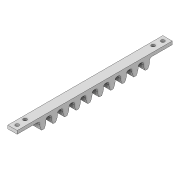
# Autodesk Inventor part: rack6mm-v2-bottom
Saved by Autodesk Inventor 2020 (Build 240168000, 168)
## iProperties
Created: 2021-06-14
Part Number: rack6mm-v2-bottom
Material: Generic
Document SubType Name: Modeling
Designer: Aidan Lee
Density: 1 g/cm^3
Appearance: Default
Author: Aidan Lee
Autodesk Inventor part; units mm, degrees
ref_plane "YZ Plane" through (0, 0, 0) normal (1, 0, 0) x (0, 1, 0)
sketch "Sketch2" plane through (0, 0, 0) normal (0, 0, 1) x (1, 0, 0)
  line L0 (-32.0857, 0) -> (0, 0)
  line L1 (0, 0) -> (0, 19.635)
  line L2 (0, 19.635) -> (-32.0857, 19.635)
  spline S0 degree 3 poles (-32.0857, 19.635) (-32.0786, 19.6019) (-32.0585, 19.4984) (-32.0378, 19.3226) (-32.0222, 19.1083) (-32.0293, 18.8935) (-32.0484, 18.6795) (-32.102, 18.3981) (-32.1765, 18.0482) (-32.2416, 17.6965) (-32.2997, 17.416) (-32.364, 17.211) (-32.4396, 17.0099) (-32.536, 16.8179) (-32.6409, 16.6304) (-32.7641, 16.4543) (-32.8983, 16.2866) (-33.043, 16.1278) (-33.201, 15.9822) (-33.3669, 15.8459) (-33.5414, 15.7205) (-33.7857, 15.5713) (-34.1055, 15.4094) (-34.509, 15.2608) (-34.9249, 15.1525) (-35.3479, 15.078) (-35.7753, 15.0341) (-36.2047, 15.0215) (-36.6341, 15.0313) (-37.0623, 15.0646) (-37.3462, 15.1014) (-37.4881, 15.1198) knots -0.847201 -0.847201 -0.847201 -0.847201 -0.83705 -0.815587 -0.794126 -0.772659 -0.751201 -0.729734 -0.686802 -0.64387 -0.622403 -0.600945 -0.579478 -0.558017 -0.536554 -0.515088 -0.49363 -0.472163 -0.450698 -0.429238 -0.407769 -0.386302 -0.343394 -0.300476 -0.257562 -0.214646 -0.17172 -0.12879 -0.085861 -0.04293 0 0 0 0
  spline S1 degree 3 poles (-37.4881, 15.1198) (-37.594, 15.1249) (-37.8057, 15.1352) (-38.2295, 15.119) (-38.7575, 15.0717) (-39.3865, 14.9771) (-40.0103, 14.8535) (-40.6285, 14.7043) (-41.2408, 14.5326) (-41.847, 14.3405) (-42.4469, 14.1297) (-43.0405, 13.9015) (-43.6276, 13.6572) (-44.2081, 13.3977) (-44.782, 13.1239) (-45.3493, 12.8367) (-45.9097, 12.5363) (-46.4639, 12.2246) (-46.8275, 12.0066) (-47.0092, 11.8976) knots -1.017256 -1.017256 -1.017256 -1.017256 -0.985476 -0.953687 -0.890117 -0.826542 -0.762964 -0.699386 -0.635807 -0.572227 -0.508647 -0.445066 -0.381486 -0.317905 -0.254324 -0.190743 -0.127162 -0.063581 0 0 0 0
  arc A0 (-47.0092, 11.8976) -> (-47.0092, 7.7374) centre (9.2023, 9.8175) ccw
  spline S2 degree 3 poles (-47.0092, 7.7374) (-46.8275, 7.6284) (-46.4639, 7.4104) (-45.9097, 7.0987) (-45.3493, 6.7983) (-44.782, 6.5111) (-44.2081, 6.2373) (-43.6276, 5.9778) (-43.0405, 5.7335) (-42.4469, 5.5053) (-41.847, 5.2945) (-41.2408, 5.1024) (-40.6285, 4.9307) (-40.0103, 4.7815) (-39.3865, 4.6579) (-38.7575, 4.5633) (-38.2295, 4.516) (-37.8057, 4.4998) (-37.594, 4.5101) (-37.4881, 4.5152) knots -1.017256 -1.017256 -1.017256 -1.017256 -0.953675 -0.890094 -0.826513 -0.762932 -0.699351 -0.63577 -0.572189 -0.508609 -0.445029 -0.381449 -0.31787 -0.254291 -0.190714 -0.127139 -0.063568 -0.03178 0 0 0 0
  spline S3 degree 3 poles (-37.4881, 4.5152) (-37.3462, 4.5336) (-37.0623, 4.5704) (-36.6341, 4.6037) (-36.2047, 4.6135) (-35.7753, 4.6009) (-35.3479, 4.557) (-34.9249, 4.4825) (-34.509, 4.3742) (-34.1055, 4.2256) (-33.7857, 4.0637) (-33.5414, 3.9145) (-33.3669, 3.7891) (-33.201, 3.6528) (-33.043, 3.5072) (-32.8983, 3.3484) (-32.7641, 3.1807) (-32.6409, 3.0046) (-32.536, 2.8171) (-32.4396, 2.6251) (-32.364, 2.424) (-32.2997, 2.219) (-32.2416, 1.9385) (-32.1765, 1.5868) (-32.102, 1.2369) (-32.0484, 0.9555) (-32.0293, 0.7415) (-32.0222, 0.5267) (-32.0378, 0.3124) (-32.0585, 0.1366) (-32.0786, 0.0331) (-32.0857, 0) knots -1.373604 -1.373604 -1.373604 -1.373604 -1.330674 -1.287743 -1.244814 -1.201884 -1.158958 -1.116042 -1.073128 -1.03021 -0.987302 -0.965835 -0.944366 -0.922906 -0.901441 -0.879974 -0.858516 -0.83705 -0.815587 -0.794126 -0.772659 -0.751201 -0.729734 -0.686802 -0.64387 -0.622403 -0.600945 -0.579478 -0.558017 -0.536554 -0.526403 -0.526403 -0.526403 -0.526403
  constraints: 6 end point, 2 centre point, 2 point on circle, 16 other
extrude "Extrusion1" add sketch "Sketch2" along normal blind 16
pattern_linear "Rectangular Pattern1" count 10 spacing 19.635 along (0, 1, 0) of "Extrusion1"
sketch "Sketch5" plane through (-32.0857, 0, 0) normal (0, -1, 0) x (1, 0, 0)
  line L0 (32.0857, 0) -> (32.0857, 16) projected
  line L1 (0, 16) -> (32.0857, 16) projected
  line L2 (0, 0) -> (32.0857, 0) projected
  line L3 (0, 0) -> (0, 16) projected
  line L4 (0, 16) -> (8, 16)
  line L5 (8, 16) -> (8, 0) construction
  line L6 (8, 0) -> (0, 0)
  line L7 (0, 0) -> (0, 16)
  line L8 (8, 16) -> (10.5, 16)
  line L9 (10.5, 16) -> (10.5, 10.5)
  line L10 (10.5, 10.5) -> (8, 10.5)
  line L11 (8, 10.5) -> (8, 16) construction
  line L12 (8, 2.5) -> (10.5, 2.5)
  line L13 (10.5, 2.5) -> (10.5, 0)
  line L14 (10.5, 0) -> (8, 0)
  line L15 (8, 0) -> (8, 2.5) construction
  line L16 (8, 9.5) -> (37, 9.5) construction
  line L17 (37, 9.5) -> (37, 3.5) construction
  line L18 (37, 3.5) -> (8, 3.5) construction
  line L19 (8, 3.5) -> (8, 9.5) construction
  line L20 (8, 10.5) -> (8, 2.5)
  line L21 (34.5, 15.5) -> (10.5, 15.5) construction
  line L22 (10.5, 15.5) -> (10.5, 0.5) construction
  line L23 (10.5, 0.5) -> (34.5, 0.5) construction
  line L24 (34.5, 0.5) -> (34.5, 15.5) construction
  line L25 (41.5759, 16) -> (41.5759, 15.5) construction
  line L26 (41.5759, 0.5) -> (41.5759, 0) construction
  line L27 (25.6, 16.05) -> (19.4, 16.05) construction
  line L28 (19.4, -0.05) -> (25.6, -0.05) construction
  line L29 (25.6, -0.05) -> (25.6, 0.5) construction
  line L30 (25.6, 15.5) -> (25.6, 16.05) construction
  line L31 (19.4, 16.05) -> (19.4, 15.5) construction
  line L32 (19.4, 0.5) -> (19.4, -0.05) construction
  line L33 (25.6, 0.5) -> (25.6, 15.5) construction
  line L34 (19.4, 15.5) -> (19.4, 0.5) construction
  point P0 (9.25, 10.5)
  point P1 (9.25, 2.5)
  point P2 (8, 6.5)
  point P3 (8, 6.5)
  point P4 (22.5, 15.5)
  point P5 (22.5, 9.5)
  point P6 (22.5, -0.05)
  dimension "d15" = 8
  dimension "d16" = 8
  dimension "d18" = 6
  dimension "d19" = 29
  dimension "d20" = 24
  dimension "d21" = 6
  dimension "d22" = 3
  dimension "d23" = 2.5
  dimension "d24" = 2.5
  dimension "d30" = 5.5
  dimension "d31" = 2.5
  dimension "d64" = 6.2
  dimension "d65" = 16.1
  constraints: 62 end point, 16 parallel, 14 point on line, 7 midpoint, 7 perpendicular, 6 horizontal, 5 collinear, 3 vertical, 2 horizontal alignment, 2 vertical alignment, 1 coincident
  measures "d15" distance between parallel lines of L3 L5
  measures "d16" distance between parallel lines of L12 L10
  measures "d18" distance of L16.end L17.end
  measures "d19" distance of L16.start L16.end
  measures "d20" distance of L21.start L21.end
  measures "d21" distance between parallel lines of L16 L21
  measures "d22" distance between parallel lines of L23 L18
  measures "d23" distance between parallel lines of L5 L22
  measures "d24" distance between parallel lines of L11 L9
  measures "d30" distance of L8.end L9.end
  measures "d31" distance of L12.end L13.end
  measures "d64" distance of L27.start L27.end
  measures "d65" distance between parallel lines of L28 L27
extrude "Extrusion3" cut sketch "Sketch5" against normal through all contours L2 L13 L12 L20 L10 L9 L1 L0
sketch "Measurements" plane through (0, 0, 0) normal (0, 0, -1) x (-1, 0, 0)
  line L0 (41.7977, 19.635) -> (70.5831, 19.635) construction
  line L1 (141.7977, 176.7146) -> (141.7977, 118.484) construction
  line L2 (21.5857, 196.35) -> (21.5857, 0) projected
  line L3 (32.0857, 0) -> (21.5857, 0) projected
  circle A0 centre (91.7977, 19.635) radius 50 construction
  line L4 (41.7977, -40.4843) -> (41.7977, 79.7543) construction
  line L5 (41.7977, 19.635) -> (141.7977, 19.635) construction
  line L6 (141.7977, 19.635) -> (141.7977, 176.7146) construction
  arc A1 (41.7977, 19.635) -> (141.7977, 176.7146) centre (-31.5724, 176.7146) ccw construction
  circle A2 centre (91.7977, 176.7146) radius 50 construction
  line L7 (-14.9143, 139.9646) -> (32.0857, 139.9646) construction
  line L8 (32.0857, 139.9646) -> (32.0857, 213.4646) construction
  line L9 (32.0857, 213.4646) -> (-14.9143, 213.4646) construction
  line L10 (-14.9143, 213.4646) -> (-14.9143, 139.9646) construction
  circle A3 centre (91.7977, 176.7146) radius 5 construction
  line L11 (32.0857, 139.9646) -> (96.4406, 164.572) construction
  arc A4 (96.4406, 164.572) -> (96.4406, 188.8572) centre (91.7977, 176.7146) ccw construction
  line L12 (96.4406, 188.8572) -> (32.0857, 213.4646) construction
  line L13 (-14.9143, -17.115) -> (32.0857, -17.115) construction
  line L14 (32.0857, -17.115) -> (32.0857, 56.385) construction
  line L15 (32.0857, 56.385) -> (-14.9143, 56.385) construction
  line L16 (-14.9143, 56.385) -> (-14.9143, -17.115) construction
  circle A5 centre (91.7977, 19.635) radius 5 construction
  line L17 (32.0857, -17.115) -> (96.4406, 7.4924) construction
  arc A6 (96.4406, 7.4924) -> (96.4406, 31.7776) centre (91.7977, 19.635) ccw construction
  line L18 (96.4406, 31.7776) -> (32.0857, 56.385) construction
  line L19 (96.7977, 176.7146) -> (96.7977, 157.197) construction
  line L20 (96.7977, 19.635) -> (96.7977, 0.1424) construction
  circle A7 centre (9.5857, 201.4646) radius 14.5 construction
  line L21 (-14.9143, 176.7146) -> (-21.6792, 176.7146)
  circle A8 centre (9.5857, 151.9646) radius 14.5 construction
  point P0 (0, 0)
  point P1 (32.0857, 176.7146)
  point P2 (104.7977, 176.7146)
  point P3 (104.7977, 19.635)
  point P4 (32.0857, 19.635)
  dimension "d43" = 10
  dimension "d32" = 100
  dimension "d33" = 157.0796
  dimension "d34" = 59.712
  dimension "d36" = 73.5
  dimension "d37" = 47
  dimension "d38" = 73.5
  dimension "d39" = 47
  dimension "d41" = 8
  dimension "d44" = 17.115
  dimension "d66" = 29
  dimension "d67" = 12
  dimension "d68" = 24.5
  constraints: 40 end point, 11 point on circle, 9 vertical alignment, 7 centre point, 7 tangent, 6 parallel, 5 horizontal alignment, 5 midpoint, 5 perpendicular, 4 coincident, 4 vertical, 3 horizontal, 1 point on line, 1 symmetric about line, 5 other
  measures "d32" diameter of A0
  measures "d33" distance of L5.end L1.start
  measures "d34" horizontal distance of L3.start A0.centre
  measures "d36" distance of L9.end L7.start
  measures "d37" distance of L7.start L7.end
  measures "d38" distance of L16.start L13.start
  measures "d39" distance of L13.start L13.end
  measures "d44" distance between parallel lines of L13 L3
  measures "d66" diameter of A7
  measures "d67" distance from line of L9 A7.centre
  measures "d68" distance from line of L10 A7.centre
ref_plane "Midplane" through (-32.0857, 98.175, 0) normal (0, -1, 0) x (1, 0, 0)
sketch "Sketch10" plane through (-32.0857, 196.35, 16) normal (0, 1, 0) x (1, 0, 0)
  line L0 (0, 16) -> (0, 0) projected
  line L1 (10.5, 16) -> (0, 16) projected
  line L2 (0, 16) -> (10.5, 16)
  line L3 (10.5, 13.5) -> (10.5, 16)
  line L4 (10.5, 13.5) -> (8, 13.5) projected
  line L5 (8, 13.5) -> (10.5, 13.5)
  line L6 (8, 13.5) -> (8, 5.5) projected
  line L7 (8, 5.5) -> (8, 13.5)
  line L8 (8, 5.5) -> (10.5, 5.5) projected
  line L9 (10.5, 5.5) -> (8, 5.5)
  line L10 (10.5, 5.5) -> (10.5, 0)
  line L11 (10.5, 0) -> (0, 0)
  line L12 (0, 0) -> (0, 16)
  point P0 (32.0857, 16)
  constraints: 16 end point, 3 vertical, 2 collinear, 2 perpendicular, 1 horizontal
extrude "Extra" add sketch "Sketch10" along normal blind 18
sketch "Sketch11" plane through (-32.0857, 214.35, 16) normal (0, 1, 0) x (1, 0, 0)
  line L0 (0, 16) -> (15.5, 16)
  line L1 (15.5, 16) -> (15.5, 0)
  line L2 (15.5, 0) -> (0, 0)
  line L3 (0, 0) -> (0, 16)
  line L4 (0, 0) -> (10.5, 0) projected
  line L5 (10.5, 16) -> (0, 16) projected
  line L6 (10.5, 0) -> (10.5, 5.5) projected
  line L7 (0, 16) -> (0, 0) projected
  point P0 (32.0857, 16)
  dimension "d63" = 5
  constraints: 8 end point, 3 collinear, 2 parallel, 1 horizontal, 1 perpendicular
  measures "d63" distance between parallel lines of L1 L6
extrude "Bracket" add sketch "Sketch11" along normal blind 16
sketch "Sketch13" plane through (-16.5857, 214.35, 16) normal (1, 0, 0) x (0, 0, -1)
  circle A0 centre (8, 8) radius 5.865
  line L0 (16, 0) -> (16, 16) projected
  line L1 (0, 16) -> (16, 16) projected
  point P0 (16, -214.35)
  point P1 (16, 8)
  point P2 (8, 16)
  dimension "d69" = 11.73
  constraints: 2 midpoint, 1 centre point, 1 horizontal alignment, 1 vertical alignment
  measures "d69" diameter of A0
hole "Hole1" at (-16.5857, 222.35, 8) direction (-1, 0, 0) diameter 6 end through all countersink diameter 11.73 countersink angle 90
fillet "Fillet2" radius 2 3 edges at (-21.5857, 214.35, 1.25) (-24.0857, 214.35, 6.5) (-21.5857, 214.35, 13.25)
fillet "Fillet3" radius 1 1 edges at (-16.5857, 214.35, 8)
mirror "Mirror3" about plane through (-32.0857, 98.175, 0) normal (0, -1, 0) of "Fillet2", "Fillet3", "Hole1", "Bracket", "Extra"
ref_plane "Work Plane2" through (-26.5857, 212.35, 16) normal (1, 0, 0) x (0, 0, -1)
sketch "Sketch14" plane through (-26.5857, 212.35, 16) normal (1, 0, 0) x (0, 0, -1)
  line L0 (26.8583, 24.8606) -> (-9.9213, 24.8606)
  line L1 (-9.9213, 24.8606) -> (-9.9213, -261.2458)
  line L2 (-9.9213, -261.2458) -> (26.8583, -261.2458)
  line L3 (26.8583, -261.2458) -> (26.8583, 24.8606)
  point P0 (16, -212.35)
  constraints: 8 end point, 2 parallel, 1 horizontal, 1 perpendicular
extrude "Extrusion7" cut sketch "Sketch14" along normal through all
sketch "Sketch15" plane through (-26.5857, 212.35, 16) normal (1, 0, 0) x (0, 0, -1)
  circle A0 centre (6.5, -223.35) radius 3
  line L0 (-43.7239, -114.175) -> (-75.2168, -114.175)
  line L1 (-31.0608, 18) -> (-31.0608, -246.35) construction
  circle A1 centre (6.5, -5) radius 3
  line L2 (16, -246.35) -> (0, -246.35) construction
  line L3 (0, -246.35) -> (0, 18) projected
  line L4 (16, 18) -> (16, -246.35) projected
  point P0 (16, -212.35)
  point P1 (-31.0608, -114.175)
  dimension "d82" = 6
  dimension "d83" = 23
  dimension "d87" = 9.5
  constraints: 4 end point, 3 horizontal alignment, 2 centre point, 1 horizontal, 1 midpoint, 1 symmetric about line, 1 vertical, 1 other
  measures "d82" diameter of A0
  measures "d83" distance from line of L2 A0.centre
  measures "d87" distance from line of L4 A0.centre
extrude "Extrusion8" cut sketch "Sketch15" against normal through all
body "Solid1"
